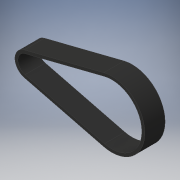
# Autodesk Inventor part: Belt
Saved by Autodesk Inventor 2019.3 (Build 233278000, 278)
## iProperties
Created: 2019-03-02
Part Number: Belt
Material: Rubber, Silicone
Document SubType Name: Modeling
Designer: Petar
Density: 1.25 g/cm^3
Appearance: Rubber - Black
Mass: 9.72075 g
Surface Area: 81.0652 cm^2
Volume: 7.7766 cm^3
Author: Petar
Autodesk Inventor part; units mm, degrees
ref_plane "YZ Plane" through (0, 0, 0) normal (1, 0, 0) x (0, 1, 0)
ref_plane "XZ Plane" through (0, 0, 0) normal (0, 1, 0) x (-1, 0, 0)
ref_plane "XY Plane" through (0, 0, 0) normal (0, 0, 1) x (1, 0, 0)
sketch "Sketch1" plane through (0, 0, 0) normal (0, 0, 1) x (1, 0, 0)
  circle A0 centre (0, 0) radius 7.64 construction
  line L0 (0, 0) -> (62.5, 0) construction
  arc A1 (-1.6967, 6.7294) -> (-1.6967, -6.7294) centre (0, 0) ccw
  arc A2 (9.14, 0) -> (4.0706, 8.1835) centre (0, 0) ccw construction
  circle A3 centre (62.5, 0) radius 22.92 construction
  arc A4 (57.0677, -21.5457) -> (57.0677, 21.5457) centre (62.5, 0) ccw
  arc A5 (38.08, 0) -> (47.2455, -19.0692) centre (62.5, 0) ccw construction
  line L1 (-2.2345, 8.8626) -> (56.5298, 23.679)
  line L2 (-2.2345, -8.8626) -> (56.5298, -23.679)
  line L3 (-1.6967, 6.7294) -> (57.0677, 21.5457)
  line L4 (-1.6967, -6.7294) -> (57.0677, -21.5457)
  arc A6 (40.28, 0) -> (57.0677, -21.5457) centre (62.5, 0) ccw construction
  arc A7 (57.0677, 21.5457) -> (40.28, 0) centre (62.5, 0) ccw construction
  arc A8 (6.94, 0) -> (-1.6967, 6.7294) centre (0, 0) ccw construction
  arc A9 (-1.6967, -6.7294) -> (6.94, 0) centre (0, 0) ccw construction
  arc A10 (4.0706, -8.1835) -> (9.14, 0) centre (0, 0) ccw construction
  arc A11 (4.0706, 8.1835) -> (-2.2345, 8.8626) centre (0, 0) ccw construction
  arc A12 (47.2455, 19.0692) -> (38.08, 0) centre (62.5, 0) ccw construction
  arc A13 (47.2455, -19.0692) -> (56.5298, -23.679) centre (62.5, 0) ccw construction
  arc A14 (-2.2345, 8.8626) -> (-2.2345, -8.8626) centre (0, 0) ccw
  arc A15 (-2.2345, -8.8626) -> (4.0706, -8.1835) centre (0, 0) ccw construction
  arc A16 (56.5298, 23.679) -> (47.2455, 19.0692) centre (62.5, 0) ccw construction
  arc A17 (56.5298, -23.679) -> (56.5298, 23.679) centre (62.5, 0) ccw
  dimension "d0" = 15.28
  dimension "d1" = 62.5
  dimension "d3" = 1.5
  dimension "d4" = 45.84
  dimension "d5" = 0.7
  dimension "d6" = 0.7
  dimension "d7" = 1.5
  constraints: 34 point on circle, 18 centre point, 12 tangent, 10 end point, 8 point on line, 6 coincident, 4 symmetric about line, 1 horizontal
  measures "d0" diameter of A0
  measures "d1" distance of L0.start L0.end
  measures "d3" radial gap between concentric circles of A2 A0
  measures "d4" diameter of A3
  measures "d5" radial gap between concentric circles of A1 A0
  measures "d6" radial gap between concentric circles of A4 A3
  measures "d7" radial gap between concentric circles of A3 A5
extrude "Extrusion1" add sketch "Sketch1" along normal blind 15
body "Solid1"
